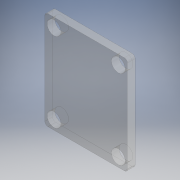
# Autodesk Inventor part: cubierta1
Saved by Autodesk Inventor 2016 (Build 200138000, 138)
## iProperties
Created: 2017-05-08
Part Number: cubierta1
Material: Polycarbonate, Smoke
Document SubType Name: Modeling
Designer: rdiaz
Density: 1.2 g/cm^3
Appearance: Polycarbonate - Clear
Author: rdiaz
Autodesk Inventor part; units mm, degrees
ref_plane "YZ Plane" through (0, 0, 0) normal (1, 0, 0) x (0, 1, 0)
ref_plane "XZ Plane" through (0, 0, 0) normal (0, 1, 0) x (-1, 0, 0)
ref_plane "XY Plane" through (0, 0, 0) normal (0, 0, 1) x (1, 0, 0)
sketch "Sketch1" plane through (0, 0, 0) normal (0, 1, 0) x (-1, 0, 0)
  line L0 (32, 27) -> (-32, 27)
  line L1 (-32, 27) -> (-32, -27)
  line L2 (-32, -27) -> (32, -27)
  line L3 (32, -27) -> (32, 27)
  point P0 (0, -27)
  point P1 (32, 0)
  point P2 (0, 0)
  dimension "d13" = 64
  dimension "d14" = 54
  constraints: 8 end point, 2 midpoint, 2 parallel, 1 horizontal, 1 horizontal alignment, 1 perpendicular, 1 vertical alignment
  measures "d13" distance between parallel lines of L3 L1
  measures "d14" distance between parallel lines of L0 L2
extrude "Extrusion1" add sketch "Sketch1" against normal blind 5
fillet "Fillet1" radius 2 4 edges at (-32, -2.5, 27) (-32, -2.5, -27) (32, -2.5, 27) (32, -2.5, -27)
sketch "Sketch2" plane through (0, -5, 0) normal (0, -1, 0) x (1, 0, 0)
  arc A0 (30, -27) -> (32, -25) centre (30, -25) ccw projected
  line L0 (32, -25) -> (32, 25) projected
  arc A1 (32, 25) -> (30, 27) centre (30, 25) ccw projected
  line L1 (30, 27) -> (-30, 27) projected
  arc A2 (-30, 27) -> (-32, 25) centre (-30, 25) ccw projected
  line L2 (-32, 25) -> (-32, -25) projected
  arc A3 (-32, -25) -> (-30, -27) centre (-30, -25) ccw projected
  line L3 (-30, -27) -> (30, -27) projected
  line L4 (20, 15) -> (-20, 15) construction
  line L5 (-20, 15) -> (-20, -15) construction
  line L6 (-20, -15) -> (20, -15) construction
  line L7 (20, -15) -> (20, 15) construction
  line L8 (-32, 27) -> (32, 27) construction
  line L9 (32, 27) -> (32, -27) construction
  line L10 (32, -27) -> (-32, -27) construction
  line L11 (-32, -27) -> (-32, 27) construction
  line L12 (-32, 27) -> (-20, 15) construction
  line L13 (-32, -27) -> (-20, -15) construction
  line L14 (32, -27) -> (20, -15) construction
  line L15 (32, 27) -> (20, 15) construction
  point P0 (0, 0)
  point P1 (0, 0)
  point P2 (0, -15)
  point P3 (20, 0)
  point P4 (0, 27)
  point P5 (32, 0)
  point P6 (-32, 0)
  point P7 (0, -27)
  point P8 (-26, -21)
  point P9 (26, -21)
  point P10 (26, 21)
  point P11 (-26, 21)
  dimension "d15" = 40
  dimension "d16" = 30
  dimension "d19" = 12
  dimension "d20" = 12
  dimension "d21" = 64
  dimension "d22" = 54
  dimension "d23" = 6
  constraints: 24 end point, 10 midpoint, 4 parallel, 4 perpendicular, 3 horizontal alignment, 3 vertical alignment, 2 horizontal, 1 point on line, 1 tangent
  measures "d15" distance of L5.end L6.end
  measures "d16" distance of L6.end L4.start
  measures "d19" distance between parallel lines of L1 L4
  measures "d20" distance between parallel lines of L2 L5
  measures "d21" distance between parallel lines of L9 L11
  measures "d22" distance between parallel lines of L3 L8
  measures "d23" distance from line of point (26, -21) L0
hole "Hole1" at (-26, -5, -21) at (26, -5, -21) at (26, -5, 21) at (-26, -5, 21) direction (0, 1, 0) diameter 9 end through all
body "Solid1"
